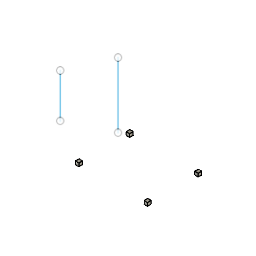
p3-caps (Autodesk Fusion 360 design; units mm, degrees)
part number: 2025-10-23-22-53-42-318
Autodesk Fusion 360 part; units mm, degrees
sketch "Sketch1" plane through (60, 0, 0) normal (1, 0, 0) x (0, 1, 0)
  line L0 (-53.75, 184.5) -> (-53.75, 192.5)
  line L1 (-53.75, 192.5) -> (-61.75, 192.5)
  spline S0 degree 5 poles (-61.75, 184.5) (-61.8258, 184.66) (-61.9709, 184.98) (-62.1687, 185.46) (-62.3919, 186.1) (-62.5991, 186.9) (-62.7279, 187.7) (-62.772, 188.5) (-62.7279, 189.3) (-62.5991, 190.1) (-62.3919, 190.9) (-62.1687, 191.54) (-61.9709, 192.02) (-61.8258, 192.34) (-61.75, 192.5) knots 0 0 0 0 0 0 0.1 0.2 0.3 0.4 0.5 0.6 0.7 0.8 0.9 1 1 1 1 1 1
  line L2 (-61.75, 184.5) -> (-53.75, 184.5)
  circle A0 centre (65.0332, 72.6084) radius 9
  line L3 (10, 205.7433) -> (10, 210)
  line L4 (10, 210) -> (5.9808, 194.0373)
  line L5 (5.9808, 194.0373) -> (-5.9808, 194.0373)
  line L6 (-5.9808, 194.0373) -> (-10, 210)
  line L7 (-10, 210) -> (-10, 205.7433)
  line L8 (-10, 205.7433) -> (-11, 205.7433)
  line L9 (-11, 205.7433) -> (-11, 210)
  line L10 (-11, 210) -> (-82.5556, 210)
  line L11 (-82.5556, 210) -> (-82.5556, 110)
  line L12 (-82.5556, 110) -> (-64.9229, 10)
  line L13 (-64.9229, 10) -> (64.9229, 10)
  line L14 (64.9229, 10) -> (82.5556, 110)
  line L15 (82.5556, 110) -> (82.5556, 210)
  line L16 (82.5556, 210) -> (11, 210)
  line L17 (11, 210) -> (11, 205.7433)
  line L18 (11, 205.7433) -> (10, 205.7433)
  line L19 (61.75, 184.5) -> (53.75, 184.5)
  line L20 (53.75, 184.5) -> (53.75, 35.5)
  line L21 (53.75, 35.5) -> (61.75, 35.5)
  spline S1 degree 5 poles (61.75, 35.5) (61.8258, 35.34) (61.9709, 35.02) (62.1687, 34.54) (62.3919, 33.9) (62.5991, 33.1) (62.7279, 32.3) (62.772, 31.5) (62.7279, 30.7) (62.5991, 29.9) (62.3919, 29.1) (62.1687, 28.46) (61.9709, 27.98) (61.8258, 27.66) (61.75, 27.5) knots 0 0 0 0 0 0 0.1 0.2 0.3 0.4 0.5 0.6 0.7 0.8 0.9 1 1 1 1 1 1
  line L22 (61.75, 27.5) -> (-61.75, 27.5)
  spline S2 degree 5 poles (-61.75, 27.5) (-61.8258, 27.66) (-61.9709, 27.98) (-62.1687, 28.46) (-62.3919, 29.1) (-62.5991, 29.9) (-62.7279, 30.7) (-62.772, 31.5) (-62.7279, 32.3) (-62.5991, 33.1) (-62.3919, 33.9) (-62.1687, 34.54) (-61.9709, 35.02) (-61.8258, 35.34) (-61.75, 35.5) knots 0 0 0 0 0 0 0.1 0.2 0.3 0.4 0.5 0.6 0.7 0.8 0.9 1 1 1 1 1 1
  line L23 (-61.75, 35.5) -> (-53.75, 35.5)
  line L24 (-53.75, 35.5) -> (-53.75, 184.5)
  line L25 (-53.75, 184.5) -> (-61.75, 184.5)
  spline S3 degree 5 poles (-61.75, 184.5) (-61.8258, 184.66) (-61.9709, 184.98) (-62.1687, 185.46) (-62.3919, 186.1) (-62.5991, 186.9) (-62.7279, 187.7) (-62.772, 188.5) (-62.7279, 189.3) (-62.5991, 190.1) (-62.3919, 190.9) (-62.1687, 191.54) (-61.9709, 192.02) (-61.8258, 192.34) (-61.75, 192.5) knots 0 0 0 0 0 0 0.1 0.2 0.3 0.4 0.5 0.6 0.7 0.8 0.9 1 1 1 1 1 1
  line L26 (-61.75, 192.5) -> (61.75, 192.5)
  spline S4 degree 5 poles (61.75, 192.5) (61.8258, 192.34) (61.9709, 192.02) (62.1687, 191.54) (62.3919, 190.9) (62.5991, 190.1) (62.7279, 189.3) (62.772, 188.5) (62.7279, 187.7) (62.5991, 186.9) (62.3919, 186.1) (62.1687, 185.46) (61.9709, 184.98) (61.8258, 184.66) (61.75, 184.5) knots 0 0 0 0 0 0 0.1 0.2 0.3 0.4 0.5 0.6 0.7 0.8 0.9 1 1 1 1 1 1
  line L27 (53.75, 184.5) -> (53.75, 192.5)
  constraint coincident L19.end L20.start
  constraint coincident L26 L27.end
  constraint perpendicular L26 L27
extrude "Extrude1" add sketch "Sketch1" along normal blind 10 contours L0 L1 S0 L2 L25 S3 L26 makes body 1
move_face "OffsetFaces1" offset -2 1 faces at (60, -56.7485, 188.4156) on bodies 1
fillet "Fillet1" radius 0.5 1 faces at (62, -56.75, 188.5071) on bodies 1
pattern_linear "R-Pattern1" count 2 spacing 157 along (0, 0, -1) of bodies 1 makes body 2
extrude "Extrude2" add sketch "Sketch1" along normal blind 10 separate body contours L19 L26 S4 L27 makes body 3
move_face "OffsetFaces2" offset -2 1 faces at (60, 56.7485, 188.5844) on bodies 3
fillet "Fillet2" radius 0.5 1 faces at (62, 56.75, 188.4929) on bodies 3
pattern_linear "R-Pattern2" count 2 spacing 157 along (0, 0, -1) of bodies 3 makes body 4
move_body "Move1" bodies 2 3 1 4 to x (0, 0, 1) y (0, 1, 0) z (-1, 0, 0) at (265.6249, 15.2855, -38.5285)
